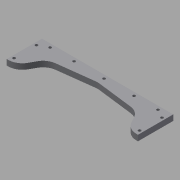
# Autodesk Inventor part: segment0c
Saved by Autodesk Inventor 2013 (Build 170138000, 138)
## iProperties
Created: 2015-09-21
Part Number: segment0c
Material: Generic
Document SubType Name: Modeling
Designer: Masta
Density: 1 g/cm^3
Author: Masta
Autodesk Inventor part; units mm, degrees
ref_plane "YZ Plane" through (0, 0, 0) normal (1, 0, 0) x (0, 1, 0)
ref_plane "XZ Plane" through (0, 0, 0) normal (0, 1, 0) x (-1, 0, 0)
ref_plane "XY Plane" through (0, 0, 0) normal (0, 0, 1) x (1, 0, 0)
sketch "Sketch1" plane through (0, 0, 0) normal (0, 0, 1) x (1, 0, 0)
  line L0 (-3.5, 6) -> (-3.5, -50) construction
  line L1 (-3.5, -50) -> (0, -50) construction
  line L2 (0, -50) -> (0, 6) construction
  line L3 (-3.5, 6) -> (0, 6) construction
  line L4 (0, 0) -> (85, 0) construction
  line L5 (85, 0) -> (85, 5) construction
  line L6 (0, 5) -> (85, 5) construction
  line L7 (0, 0) -> (0, 5) construction
  line L8 (88.5, 6) -> (88.5, -50) construction
  line L9 (88.5, 6) -> (85, 6) construction
  line L10 (85, -50) -> (85, 6) construction
  line L11 (88.5, -50) -> (85, -50) construction
  line L12 (-4, 5) -> (42.5, 5)
  line L13 (42.5, 5) -> (42.5, -2)
  line L14 (42.5, -2) -> (10.6869, -5.951)
  line L15 (10.6869, -5.951) -> (3, -20)
  line L16 (3, -20) -> (-4, -20)
  line L17 (-4, -20) -> (-4, 5)
  line L18 (0, 2.5) -> (42.5, 2.5) construction
  line L19 (-2, 5) -> (-2, -20) construction
  point P0 (4.2678, 2.5)
  point P1 (21.25, 2.5)
  point P2 (-2, -0.9091)
  point P3 (-2, -16.8032)
  dimension "d0" = 4
  dimension "d1" = 25
  dimension "d2" = 7
  dimension "d3" = 7
  dimension "d7" = 2
  constraints: 16 end point, 6 point on line, 5 perpendicular, 3 midpoint, 1 coincident
  measures "d0" distance from line of L12.start L2
  measures "d1" distance of L16.end L12.start
  measures "d2" distance of L15.end L16.end
  measures "d3" distance of L12.end L13.end
  measures "d7" distance between parallel lines of L17 L19
extrude "Extrusion1" add sketch "Sketch1" along normal blind 4
sketch "Sketch2" plane through (0, 0, 4) normal (0, 0, 1) x (1, 0, 0)
  point P0 (0, 0)
  point P1 (42.5, 2.5)
  point P2 (42.5, 2.5)
  point P3 (21.25, 2.5)
  point P4 (4.2678, 2.5)
  point P5 (-2, -0.9091)
  point P6 (-2, -16.8032)
hole "Hole1" at (42.5, 2.5, 4) at (21.25, 2.5, 4) at (4.2678, 2.5, 4) at (-2, -0.9091, 4) at (-2, -16.8032, 4) direction (0, 0, -1) diameter 2 end through all
mirror "Mirror1" about plane through (42.5, -2, 0) normal (1, 0, 0)
fillet "Fillet1" radius 10 5 edges at (3, -20, 2) (10.6869, -5.951, 2) (42.5, -2, 2) (74.3131, -5.951, 2) (82, -20, 2)
body "Solid1"
